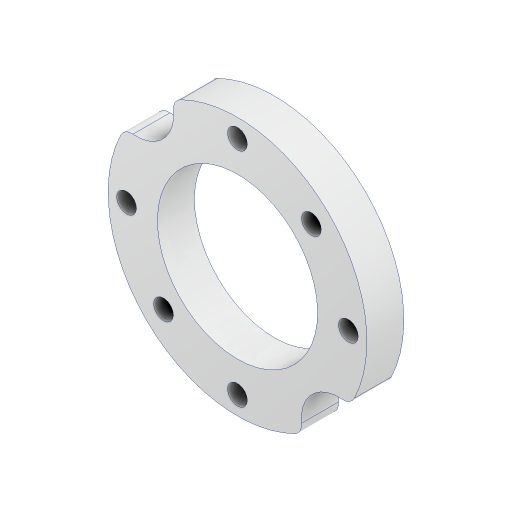
# Autodesk Inventor part: 큰기어 와셔
Saved by Autodesk Inventor 2023 (Build 270158000, 158)
## iProperties
Created: 2022-10-19
Part Number: 큰기어 와셔
Material: 알루미늄 6061
Document SubType Name: Modeling
Designer: PARK
Density: 2.7 g/cm^3
Appearance: 알루미늄 - 평지
Author: PARK
Autodesk Inventor part; units mm, degrees
ref_plane "YZ Plane" through (0, 0, 0) normal (1, 0, 0) x (0, 1, 0)
ref_plane "XZ Plane" through (0, 0, 0) normal (0, 1, 0) x (-1, 0, 0)
ref_plane "작업 평면1" through (168.9405, 113.6809, -210.8653) normal (0, 0, 1) x (-0.7019406, -0.7122354, 0)
sketch "스케치1" plane through (168.9405, 113.6809, -210.8653) normal (0, 0, 1) x (-0.7019406, -0.7122354, 0)
  circle A0 centre (0, -25.2484) radius 3 projected
  circle A1 centre (0, -2.2484) radius 13 projected
  circle A2 centre (-12.6349, 10.5718) radius 1.6 projected
  circle A3 centre (12.6349, -15.0687) radius 1.6 projected
  circle A4 centre (0.1235, 14.7217) radius 1.6 projected
  circle A5 centre (-0.1235, -19.2186) radius 1.6 projected
  circle A6 centre (-16.9701, -2.1249) radius 1.6 projected
  circle A7 centre (16.9701, -2.372) radius 1.6 projected
  circle A8 centre (12.8202, 10.3865) radius 1.6 projected
  circle A9 centre (-12.8202, -14.8834) radius 1.6 projected
  circle A10 centre (0, 20.7516) radius 3 projected
  arc A11 (-2.0317, -50.1272) -> (-0.57, -54.2453) centre (7.4248, -49.0892) ccw projected
  line L0 (0.57, -54.2453) -> (-0.57, -54.2453) projected
  arc A12 (0.57, -54.2453) -> (2.0317, -50.1272) centre (-7.4248, -49.0892) ccw projected
  arc A13 (2.5023, -49.6825) -> (2.0317, -50.1272) centre (2.5287, -50.1818) ccw projected
  arc A14 (2.5023, -49.6825) -> (3.4624, -49.6221) centre (0, -2.2484) ccw projected
  arc A15 (3.9852, -50.0043) -> (3.4624, -49.6221) centre (3.4989, -50.1207) ccw projected
  arc A16 (3.9852, -50.0043) -> (5.9514, -53.9067) centre (13.237, -47.7893) ccw projected
  line L1 (7.0824, -53.7639) -> (5.9514, -53.9067) projected
  arc A17 (7.0824, -53.7639) -> (8.0165, -49.4951) centre (-1.4956, -49.6504) ccw projected
  arc A18 (8.4277, -48.9948) -> (8.0165, -49.4951) centre (8.5164, -49.4869) ccw projected
  arc A19 (8.4277, -48.9948) -> (9.3726, -48.8146) centre (0, -2.2484) ccw projected
  arc A20 (9.9391, -49.1283) -> (9.3726, -48.8146) centre (9.4713, -49.3047) ccw projected
  arc A21 (9.9391, -49.1283) -> (12.379, -52.7535) centre (18.8404, -45.7711) ccw projected
  line L2 (13.4832, -52.47) -> (12.379, -52.7535) projected
  arc A22 (13.4832, -52.47) -> (13.8748, -48.1178) centre (4.4572, -49.4641) ccw projected
  arc A23 (14.2201, -47.5699) -> (13.8748, -48.1178) centre (14.3698, -48.047) ccw projected
  arc A24 (14.2201, -47.5699) -> (15.135, -47.2727) centre (0, -2.2484) ccw projected
  arc A25 (15.7364, -47.5129) -> (15.135, -47.2727) centre (15.2943, -47.7466) ccw projected
  arc A26 (15.7364, -47.5129) -> (18.6114, -50.8037) centre (24.1467, -43.0666) ccw projected
  line L3 (19.6713, -50.3841) -> (18.6114, -50.8037) projected
  arc A27 (19.6713, -50.3841) -> (19.5144, -46.0171) centre (10.3398, -48.5331) ccw projected
  arc A28 (19.7883, -45.4303) -> (19.5144, -46.0171) centre (19.9966, -45.8849) ccw projected
  arc A29 (19.7883, -45.4303) -> (20.6587, -45.0207) centre (0, -2.2484) ccw projected
  arc A30 (21.2854, -45.1837) -> (20.6587, -45.0207) centre (20.8762, -45.471) ccw projected
  arc A31 (21.2854, -45.1837) -> (24.5502, -48.0882) centre (29.0721, -39.7184) ccw projected
  line L4 (25.5492, -47.539) -> (24.5502, -48.0882) projected
  arc A32 (25.5492, -47.539) -> (24.8461, -43.2262) centre (16.0593, -46.8722) ccw projected
  arc A33 (25.0443, -42.6097) -> (24.8461, -43.2262) centre (25.308, -43.0345) ccw projected
  arc A34 (25.0443, -42.6097) -> (25.8566, -42.0942) centre (0, -2.2484) ccw projected
  arc A35 (26.4988, -42.1774) -> (25.8566, -42.0942) centre (26.1288, -42.5137) ccw projected
  arc A36 (26.4988, -42.1774) -> (30.1019, -44.6498) centre (33.5391, -35.7792) ccw projected
  line L5 (31.0241, -43.9798) -> (30.1019, -44.6498) projected
  arc A37 (31.0241, -43.9798) -> (29.7861, -39.789) centre (21.5255, -44.5076) ccw projected
  arc A38 (29.9055, -39.1525) -> (29.7861, -39.789) centre (30.2203, -39.541) ccw projected
  arc A39 (29.9055, -39.1525) -> (30.6467, -38.5393) centre (0, -2.2484) ccw projected
  arc A40 (31.2943, -38.5413) -> (30.6467, -38.5393) centre (30.9693, -38.9213) ccw projected
  arc A41 (31.2943, -38.5413) -> (35.1788, -40.5427) centre (37.4772, -31.3112) ccw projected
  line L6 (36.0098, -39.7623) -> (35.1788, -40.5427) projected
  arc A42 (36.0098, -39.7623) -> (34.2563, -35.7598) centre (26.6522, -41.4765) ccw projected
  arc A43 (34.295, -35.1134) -> (34.2563, -35.7598) centre (34.656, -35.4593) ccw projected
  arc A44 (34.295, -35.1134) -> (34.9535, -34.4121) centre (0, -2.2484) ccw projected
  arc A45 (35.5962, -34.333) -> (34.9535, -34.4121) centre (35.3214, -34.7507) ccw projected
  arc A46 (35.5962, -34.333) -> (39.7009, -35.8317) centre (40.8242, -26.3849) ccw projected
  line L7 (40.4276, -34.9533) -> (39.7009, -35.8317) projected
  arc A47 (40.4276, -34.9533) -> (38.1863, -31.2021) centre (31.3586, -37.8268) ccw projected
  arc A48 (38.1436, -30.5559) -> (38.1863, -31.2021) centre (38.5451, -30.8539) ccw projected
  arc A49 (38.1436, -30.5559) -> (38.7091, -29.7777) centre (0, -2.2484) ccw projected
  arc A50 (39.3368, -29.6186) -> (38.7091, -29.7777) centre (39.1165, -30.0674) ccw projected
  arc A51 (39.3368, -29.6186) -> (43.597, -30.591) centre (43.5274, -21.078) ccw projected
  line L8 (44.2078, -29.6285) -> (43.597, -30.591) projected
  arc A52 (44.2078, -29.6285) -> (41.514, -26.1878) centre (35.5705, -33.616) ccw projected
  arc A53 (41.3907, -25.5521) -> (41.514, -26.1878) centre (41.8264, -25.7974) ccw projected
  arc A54 (41.3907, -25.5521) -> (41.8542, -24.7091) centre (0, -2.2484) ccw projected
  arc A55 (42.457, -24.4725) -> (41.8542, -24.7091) centre (42.2947, -24.9455) ccw projected
  arc A56 (42.457, -24.4725) -> (46.8055, -24.9034) centre (45.5441, -15.4741) ccw projected
  line L9 (47.2909, -23.8719) -> (46.8055, -24.9034) projected
  arc A57 (47.2909, -23.8719) -> (44.1871, -20.7959) centre (39.2214, -28.9105) ccw projected
  arc A58 (43.985, -20.1807) -> (44.1871, -20.7959) centre (44.4481, -20.3694) ccw projected
  arc A59 (43.985, -20.1807) -> (44.3392, -19.2862) centre (0, -2.2484) ccw projected
  arc A60 (44.9076, -18.976) -> (44.3392, -19.2862) centre (44.8059, -19.4656) ccw projected
  arc A61 (44.9076, -18.976) -> (49.2758, -18.8585) centre (46.8426, -9.6616) ccw projected
  line L10 (49.6281, -17.7743) -> (49.2758, -18.8585) projected
  arc A62 (49.6281, -17.7743) -> (46.1633, -15.1116) centre (42.2538, -23.7845) ccw projected
  arc A63 (45.8857, -14.5265) -> (46.1633, -15.1116) centre (46.3687, -14.6557) ccw projected
  arc A64 (45.8857, -14.5265) -> (46.125, -13.5947) centre (0, -2.2484) ccw projected
  arc A65 (46.65, -13.2157) -> (46.125, -13.5947) centre (46.6105, -13.7141) ccw projected
  arc A66 (46.65, -13.2157) -> (50.9691, -12.5516) centre (47.4023, -3.7322) ccw projected
  line L11 (51.1827, -11.4318) -> (50.9691, -12.5516) projected
  arc A67 (51.1827, -11.4318) -> (47.4114, -9.2243) centre (44.6198, -18.3188) ccw projected
  arc A68 (47.0627, -8.6787) -> (47.4114, -9.2243) centre (47.5581, -8.7464) ccw projected
  arc A69 (47.0627, -8.6787) -> (47.1833, -7.7243) centre (0, -2.2484) ccw projected
  arc A70 (47.6567, -7.2824) -> (47.1833, -7.7243) centre (47.68, -7.7819) ccw projected
  arc A71 (47.6567, -7.2824) -> (51.8585, -6.0822) centre (47.2145, 2.2206) ccw projected
  line L12 (51.9301, -4.9445) -> (51.8585, -6.0822) projected
  arc A72 (51.9301, -4.9445) -> (47.9119, -3.2271) centre (46.2821, -12.5998) ccw projected
  arc A73 (47.4976, -2.7294) -> (47.9119, -3.2271) centre (47.9975, -2.7345) ccw projected
  arc A74 (47.4976, -2.7294) -> (47.4976, -1.7674) centre (0, -2.2484) ccw projected
  arc A75 (47.9119, -1.2698) -> (47.4976, -1.7674) centre (47.9975, -1.7624) ccw projected
  arc A76 (47.9119, -1.2698) -> (51.9301, 0.4476) centre (46.2821, 8.1029) ccw projected
  line L13 (51.8585, 1.5853) -> (51.9301, 0.4476) projected
  arc A77 (51.8585, 1.5853) -> (47.6567, 2.7856) centre (47.2145, -6.7175) ccw projected
  arc A78 (47.1833, 3.2274) -> (47.6567, 2.7856) centre (47.68, 3.285) ccw projected
  arc A79 (47.1833, 3.2274) -> (47.0627, 4.1818) centre (0, -2.2484) ccw projected
  arc A80 (47.4114, 4.7275) -> (47.0627, 4.1818) centre (47.5581, 4.2495) ccw projected
  arc A81 (47.4114, 4.7275) -> (51.1827, 6.9349) centre (44.6198, 13.822) ccw projected
  line L14 (50.9691, 8.0547) -> (51.1827, 6.9349) projected
  arc A82 (50.9691, 8.0547) -> (46.65, 8.7188) centre (47.4023, -0.7647) ccw projected
  arc A83 (46.125, 9.0978) -> (46.65, 8.7188) centre (46.6105, 9.2173) ccw projected
  arc A84 (46.125, 9.0978) -> (45.8857, 10.0296) centre (0, -2.2484) ccw projected
  arc A85 (46.1633, 10.6147) -> (45.8857, 10.0296) centre (46.3687, 10.1589) ccw projected
  arc A86 (46.1633, 10.6147) -> (49.6281, 13.2774) centre (42.2538, 19.2876) ccw projected
  line L15 (49.2758, 14.3616) -> (49.6281, 13.2774) projected
  arc A87 (49.2758, 14.3616) -> (44.9076, 14.4792) centre (46.8426, 5.1647) ccw projected
  arc A88 (44.3392, 14.7894) -> (44.9076, 14.4792) centre (44.8059, 14.9687) ccw projected
  arc A89 (44.3392, 14.7894) -> (43.985, 15.6838) centre (0, -2.2484) ccw projected
  arc A90 (44.1871, 16.299) -> (43.985, 15.6838) centre (44.4481, 15.8726) ccw projected
  arc A91 (44.1871, 16.299) -> (47.2909, 19.375) centre (39.2214, 24.4136) ccw projected
  line L16 (46.8055, 20.4065) -> (47.2909, 19.375) projected
  arc A92 (46.8055, 20.4065) -> (42.457, 19.9757) centre (45.5441, 10.9772) ccw projected
  arc A93 (41.8542, 20.2122) -> (42.457, 19.9757) centre (42.2947, 20.4486) ccw projected
  arc A94 (41.8542, 20.2122) -> (41.3907, 21.0552) centre (0, -2.2484) ccw projected
  arc A95 (41.514, 21.6909) -> (41.3907, 21.0552) centre (41.8264, 21.3005) ccw projected
  arc A96 (41.514, 21.6909) -> (44.2078, 25.1316) centre (35.5705, 29.1191) ccw projected
  line L17 (43.597, 26.0941) -> (44.2078, 25.1316) projected
  arc A97 (43.597, 26.0941) -> (39.3368, 25.1217) centre (43.5274, 16.5811) ccw projected
  arc A98 (38.7091, 25.2808) -> (39.3368, 25.1217) centre (39.1165, 25.5706) ccw projected
  arc A99 (38.7091, 25.2808) -> (38.1436, 26.0591) centre (0, -2.2484) ccw projected
  arc A100 (38.1863, 26.7052) -> (38.1436, 26.0591) centre (38.5451, 26.357) ccw projected
  arc A101 (38.1863, 26.7052) -> (40.4276, 30.4564) centre (31.3586, 33.3299) ccw projected
  line L18 (39.7009, 31.3348) -> (40.4276, 30.4564) projected
  arc A102 (39.7009, 31.3348) -> (35.5962, 29.8361) centre (40.8242, 21.888) ccw projected
  arc A103 (34.9535, 29.9152) -> (35.5962, 29.8361) centre (35.3214, 30.2538) ccw projected
  arc A104 (34.9535, 29.9152) -> (34.295, 30.6165) centre (0, -2.2484) ccw projected
  arc A105 (34.2563, 31.2629) -> (34.295, 30.6165) centre (34.656, 30.9625) ccw projected
  arc A106 (34.2563, 31.2629) -> (36.0098, 35.2655) centre (26.6522, 36.9797) ccw projected
  line L19 (35.1788, 36.0458) -> (36.0098, 35.2655) projected
  arc A107 (35.1788, 36.0458) -> (31.2943, 34.0445) centre (37.4772, 26.8143) ccw projected
  arc A108 (30.6467, 34.0425) -> (31.2943, 34.0445) centre (30.9693, 34.4245) ccw projected
  arc A109 (30.6467, 34.0425) -> (29.9055, 34.6557) centre (0, -2.2484) ccw projected
  arc A110 (29.7861, 35.2921) -> (29.9055, 34.6557) centre (30.2203, 35.0441) ccw projected
  arc A111 (29.7861, 35.2921) -> (31.0241, 39.4829) centre (21.5255, 40.0107) ccw projected
  line L20 (30.1019, 40.153) -> (31.0241, 39.4829) projected
  arc A112 (30.1019, 40.153) -> (26.4988, 37.6805) centre (33.5391, 31.2823) ccw projected
  arc A113 (25.8566, 37.5973) -> (26.4988, 37.6805) centre (26.1288, 38.0168) ccw projected
  arc A114 (25.8566, 37.5973) -> (25.0443, 38.1128) centre (0, -2.2484) ccw projected
  arc A115 (24.8461, 38.7293) -> (25.0443, 38.1128) centre (25.308, 38.5377) ccw projected
  arc A116 (24.8461, 38.7293) -> (25.5492, 43.0422) centre (16.0593, 42.3754) ccw projected
  line L21 (24.5502, 43.5914) -> (25.5492, 43.0422) projected
  arc A117 (24.5502, 43.5914) -> (21.2854, 40.6868) centre (29.0721, 35.2215) ccw projected
  arc A118 (20.6587, 40.5238) -> (21.2854, 40.6868) centre (20.8762, 40.9741) ccw projected
  arc A119 (20.6587, 40.5238) -> (19.7883, 40.9334) centre (0, -2.2484) ccw projected
  arc A120 (19.5144, 41.5202) -> (19.7883, 40.9334) centre (19.9966, 41.388) ccw projected
  arc A121 (19.5144, 41.5202) -> (19.6713, 45.8872) centre (10.3398, 44.0363) ccw projected
  line L22 (18.6114, 46.3069) -> (19.6713, 45.8872) projected
  arc A122 (18.6114, 46.3069) -> (15.7364, 43.016) centre (24.1467, 38.5697) ccw projected
  arc A123 (15.135, 42.7758) -> (15.7364, 43.016) centre (15.2943, 43.2497) ccw projected
  arc A124 (15.135, 42.7758) -> (14.2201, 43.0731) centre (0, -2.2484) ccw projected
  arc A125 (13.8748, 43.6209) -> (14.2201, 43.0731) centre (14.3698, 43.5501) ccw projected
  arc A126 (13.8748, 43.6209) -> (13.4832, 47.9731) centre (4.4572, 44.9672) ccw projected
  line L23 (12.379, 48.2566) -> (13.4832, 47.9731) projected
  arc A127 (12.379, 48.2566) -> (9.9391, 44.6314) centre (18.8404, 41.2742) ccw projected
  arc A128 (9.3726, 44.3177) -> (9.9391, 44.6314) centre (9.4713, 44.8079) ccw projected
  arc A129 (9.3726, 44.3177) -> (8.4277, 44.4979) centre (0, -2.2484) ccw projected
  arc A130 (8.0165, 44.9982) -> (8.4277, 44.4979) centre (8.5164, 44.99) ccw projected
  arc A131 (8.0165, 44.9982) -> (7.0824, 49.267) centre (-1.4956, 45.1535) ccw projected
  line L24 (5.9514, 49.4099) -> (7.0824, 49.267) projected
  arc A132 (5.9514, 49.4099) -> (3.9852, 45.5074) centre (13.237, 43.2924) ccw projected
  arc A133 (3.4624, 45.1252) -> (3.9852, 45.5074) centre (3.4989, 45.6239) ccw projected
  arc A134 (3.4624, 45.1252) -> (2.5023, 45.1856) centre (0, -2.2484) ccw projected
  arc A135 (2.0317, 45.6304) -> (2.5023, 45.1856) centre (2.5287, 45.6849) ccw projected
  arc A136 (2.0317, 45.6304) -> (0.57, 49.7484) centre (-7.4248, 44.5923) ccw projected
  line L25 (-0.57, 49.7484) -> (0.57, 49.7484) projected
  arc A137 (-0.57, 49.7484) -> (-2.0317, 45.6304) centre (7.4248, 44.5923) ccw projected
  arc A138 (-2.5023, 45.1856) -> (-2.0317, 45.6304) centre (-2.5287, 45.6849) ccw projected
  arc A139 (-2.5023, 45.1856) -> (-3.4624, 45.1252) centre (0, -2.2484) ccw projected
  arc A140 (-3.9852, 45.5074) -> (-3.4624, 45.1252) centre (-3.4989, 45.6239) ccw projected
  arc A141 (-3.9852, 45.5074) -> (-5.9514, 49.4099) centre (-13.237, 43.2924) ccw projected
  line L26 (-7.0824, 49.267) -> (-5.9514, 49.4099) projected
  arc A142 (-7.0824, 49.267) -> (-8.0165, 44.9982) centre (1.4956, 45.1535) ccw projected
  arc A143 (-8.4277, 44.4979) -> (-8.0165, 44.9982) centre (-8.5164, 44.99) ccw projected
  arc A144 (-8.4277, 44.4979) -> (-9.3726, 44.3177) centre (0, -2.2484) ccw projected
  arc A145 (-9.9391, 44.6314) -> (-9.3726, 44.3177) centre (-9.4713, 44.8079) ccw projected
  arc A146 (-9.9391, 44.6314) -> (-12.379, 48.2566) centre (-18.8404, 41.2742) ccw projected
  line L27 (-13.4832, 47.9731) -> (-12.379, 48.2566) projected
  arc A147 (-13.4832, 47.9731) -> (-13.8748, 43.6209) centre (-4.4572, 44.9672) ccw projected
  arc A148 (-14.2201, 43.0731) -> (-13.8748, 43.6209) centre (-14.3698, 43.5501) ccw projected
  arc A149 (-14.2201, 43.0731) -> (-15.135, 42.7758) centre (0, -2.2484) ccw projected
  arc A150 (-15.7364, 43.016) -> (-15.135, 42.7758) centre (-15.2943, 43.2497) ccw projected
  arc A151 (-15.7364, 43.016) -> (-18.6114, 46.3069) centre (-24.1467, 38.5697) ccw projected
  line L28 (-19.6713, 45.8872) -> (-18.6114, 46.3069) projected
  arc A152 (-19.6713, 45.8872) -> (-19.5144, 41.5202) centre (-10.3398, 44.0363) ccw projected
  arc A153 (-19.7883, 40.9334) -> (-19.5144, 41.5202) centre (-19.9966, 41.388) ccw projected
  arc A154 (-19.7883, 40.9334) -> (-20.6587, 40.5238) centre (0, -2.2484) ccw projected
  arc A155 (-21.2854, 40.6868) -> (-20.6587, 40.5238) centre (-20.8762, 40.9741) ccw projected
  arc A156 (-21.2854, 40.6868) -> (-24.5502, 43.5914) centre (-29.0721, 35.2215) ccw projected
  line L29 (-25.5492, 43.0422) -> (-24.5502, 43.5914) projected
  arc A157 (-25.5492, 43.0422) -> (-24.8461, 38.7293) centre (-16.0593, 42.3754) ccw projected
  arc A158 (-25.0443, 38.1128) -> (-24.8461, 38.7293) centre (-25.308, 38.5377) ccw projected
  arc A159 (-25.0443, 38.1128) -> (-25.8566, 37.5973) centre (0, -2.2484) ccw projected
  arc A160 (-26.4988, 37.6805) -> (-25.8566, 37.5973) centre (-26.1288, 38.0168) ccw projected
  arc A161 (-26.4988, 37.6805) -> (-30.1019, 40.153) centre (-33.5391, 31.2823) ccw projected
  line L30 (-31.0241, 39.4829) -> (-30.1019, 40.153) projected
  arc A162 (-31.0241, 39.4829) -> (-29.7861, 35.2921) centre (-21.5255, 40.0107) ccw projected
  arc A163 (-29.9055, 34.6557) -> (-29.7861, 35.2921) centre (-30.2203, 35.0441) ccw projected
  arc A164 (-29.9055, 34.6557) -> (-30.6467, 34.0425) centre (0, -2.2484) ccw projected
  arc A165 (-31.2943, 34.0445) -> (-30.6467, 34.0425) centre (-30.9693, 34.4245) ccw projected
  arc A166 (-31.2943, 34.0445) -> (-35.1788, 36.0458) centre (-37.4772, 26.8143) ccw projected
  line L31 (-36.0098, 35.2655) -> (-35.1788, 36.0458) projected
  arc A167 (-36.0098, 35.2655) -> (-34.2563, 31.2629) centre (-26.6522, 36.9797) ccw projected
  arc A168 (-34.295, 30.6165) -> (-34.2563, 31.2629) centre (-34.656, 30.9625) ccw projected
  arc A169 (-34.295, 30.6165) -> (-34.9535, 29.9152) centre (0, -2.2484) ccw projected
  arc A170 (-35.5962, 29.8361) -> (-34.9535, 29.9152) centre (-35.3214, 30.2538) ccw projected
  arc A171 (-35.5962, 29.8361) -> (-39.7009, 31.3348) centre (-40.8242, 21.888) ccw projected
  line L32 (-40.4276, 30.4564) -> (-39.7009, 31.3348) projected
  arc A172 (-40.4276, 30.4564) -> (-38.1863, 26.7052) centre (-31.3586, 33.3299) ccw projected
  arc A173 (-38.1436, 26.0591) -> (-38.1863, 26.7052) centre (-38.5451, 26.357) ccw projected
  arc A174 (-38.1436, 26.0591) -> (-38.7091, 25.2808) centre (0, -2.2484) ccw projected
  arc A175 (-39.3368, 25.1217) -> (-38.7091, 25.2808) centre (-39.1165, 25.5706) ccw projected
  arc A176 (-39.3368, 25.1217) -> (-43.597, 26.0941) centre (-43.5274, 16.5811) ccw projected
  line L33 (-44.2078, 25.1316) -> (-43.597, 26.0941) projected
  arc A177 (-44.2078, 25.1316) -> (-41.514, 21.6909) centre (-35.5705, 29.1191) ccw projected
  arc A178 (-41.3907, 21.0552) -> (-41.514, 21.6909) centre (-41.8264, 21.3005) ccw projected
  arc A179 (-41.3907, 21.0552) -> (-41.8542, 20.2122) centre (0, -2.2484) ccw projected
  arc A180 (-42.457, 19.9757) -> (-41.8542, 20.2122) centre (-42.2947, 20.4486) ccw projected
  arc A181 (-42.457, 19.9757) -> (-46.8055, 20.4065) centre (-45.5441, 10.9772) ccw projected
  line L34 (-47.2909, 19.375) -> (-46.8055, 20.4065) projected
  arc A182 (-47.2909, 19.375) -> (-44.1871, 16.299) centre (-39.2214, 24.4136) ccw projected
  arc A183 (-43.985, 15.6838) -> (-44.1871, 16.299) centre (-44.4481, 15.8726) ccw projected
  arc A184 (-43.985, 15.6838) -> (-44.3392, 14.7894) centre (0, -2.2484) ccw projected
  arc A185 (-44.9076, 14.4792) -> (-44.3392, 14.7894) centre (-44.8059, 14.9687) ccw projected
  arc A186 (-44.9076, 14.4792) -> (-49.2758, 14.3616) centre (-46.8426, 5.1647) ccw projected
  line L35 (-49.6281, 13.2774) -> (-49.2758, 14.3616) projected
  arc A187 (-49.6281, 13.2774) -> (-46.1633, 10.6147) centre (-42.2538, 19.2876) ccw projected
  arc A188 (-45.8857, 10.0296) -> (-46.1633, 10.6147) centre (-46.3687, 10.1589) ccw projected
  arc A189 (-45.8857, 10.0296) -> (-46.125, 9.0978) centre (0, -2.2484) ccw projected
  arc A190 (-46.65, 8.7188) -> (-46.125, 9.0978) centre (-46.6105, 9.2173) ccw projected
  arc A191 (-46.65, 8.7188) -> (-50.9691, 8.0547) centre (-47.4023, -0.7647) ccw projected
  line L36 (-51.1827, 6.9349) -> (-50.9691, 8.0547) projected
  arc A192 (-51.1827, 6.9349) -> (-47.4114, 4.7275) centre (-44.6198, 13.822) ccw projected
  arc A193 (-47.0627, 4.1818) -> (-47.4114, 4.7275) centre (-47.5581, 4.2495) ccw projected
  arc A194 (-47.0627, 4.1818) -> (-47.1833, 3.2274) centre (0, -2.2484) ccw projected
  arc A195 (-47.6567, 2.7856) -> (-47.1833, 3.2274) centre (-47.68, 3.285) ccw projected
  arc A196 (-47.6567, 2.7856) -> (-51.8585, 1.5853) centre (-47.2145, -6.7175) ccw projected
  line L37 (-51.9301, 0.4476) -> (-51.8585, 1.5853) projected
  arc A197 (-51.9301, 0.4476) -> (-47.9119, -1.2698) centre (-46.2821, 8.1029) ccw projected
  arc A198 (-47.4976, -1.7674) -> (-47.9119, -1.2698) centre (-47.9975, -1.7624) ccw projected
  arc A199 (-47.4976, -1.7674) -> (-47.4976, -2.7294) centre (0, -2.2484) ccw projected
  arc A200 (-47.9119, -3.2271) -> (-47.4976, -2.7294) centre (-47.9975, -2.7345) ccw projected
  arc A201 (-47.9119, -3.2271) -> (-51.9301, -4.9445) centre (-46.2821, -12.5998) ccw projected
  line L38 (-51.8585, -6.0822) -> (-51.9301, -4.9445) projected
  arc A202 (-51.8585, -6.0822) -> (-47.6567, -7.2824) centre (-47.2145, 2.2206) ccw projected
  arc A203 (-47.1833, -7.7243) -> (-47.6567, -7.2824) centre (-47.68, -7.7819) ccw projected
  arc A204 (-47.1833, -7.7243) -> (-47.0627, -8.6787) centre (0, -2.2484) ccw projected
  arc A205 (-47.4114, -9.2243) -> (-47.0627, -8.6787) centre (-47.5581, -8.7464) ccw projected
  arc A206 (-47.4114, -9.2243) -> (-51.1827, -11.4318) centre (-44.6198, -18.3188) ccw projected
  line L39 (-50.9691, -12.5516) -> (-51.1827, -11.4318) projected
  arc A207 (-50.9691, -12.5516) -> (-46.65, -13.2157) centre (-47.4023, -3.7322) ccw projected
  arc A208 (-46.125, -13.5947) -> (-46.65, -13.2157) centre (-46.6105, -13.7141) ccw projected
  arc A209 (-46.125, -13.5947) -> (-45.8857, -14.5265) centre (0, -2.2484) ccw projected
  arc A210 (-46.1633, -15.1116) -> (-45.8857, -14.5265) centre (-46.3687, -14.6557) ccw projected
  arc A211 (-46.1633, -15.1116) -> (-49.6281, -17.7743) centre (-42.2538, -23.7845) ccw projected
  line L40 (-49.2758, -18.8585) -> (-49.6281, -17.7743) projected
  arc A212 (-49.2758, -18.8585) -> (-44.9076, -18.976) centre (-46.8426, -9.6616) ccw projected
  arc A213 (-44.3392, -19.2862) -> (-44.9076, -18.976) centre (-44.8059, -19.4656) ccw projected
  arc A214 (-44.3392, -19.2862) -> (-43.985, -20.1807) centre (0, -2.2484) ccw projected
  arc A215 (-44.1871, -20.7959) -> (-43.985, -20.1807) centre (-44.4481, -20.3694) ccw projected
  arc A216 (-44.1871, -20.7959) -> (-47.2909, -23.8719) centre (-39.2214, -28.9105) ccw projected
  line L41 (-46.8055, -24.9034) -> (-47.2909, -23.8719) projected
  arc A217 (-46.8055, -24.9034) -> (-42.457, -24.4725) centre (-45.5441, -15.4741) ccw projected
  arc A218 (-41.8542, -24.7091) -> (-42.457, -24.4725) centre (-42.2947, -24.9455) ccw projected
  arc A219 (-41.8542, -24.7091) -> (-41.3907, -25.5521) centre (0, -2.2484) ccw projected
  arc A220 (-41.514, -26.1878) -> (-41.3907, -25.5521) centre (-41.8264, -25.7974) ccw projected
  arc A221 (-41.514, -26.1878) -> (-44.2078, -29.6285) centre (-35.5705, -33.616) ccw projected
  line L42 (-43.597, -30.591) -> (-44.2078, -29.6285) projected
  arc A222 (-43.597, -30.591) -> (-39.3368, -29.6186) centre (-43.5274, -21.078) ccw projected
  arc A223 (-38.7091, -29.7777) -> (-39.3368, -29.6186) centre (-39.1165, -30.0674) ccw projected
  arc A224 (-38.7091, -29.7777) -> (-38.1436, -30.5559) centre (0, -2.2484) ccw projected
  arc A225 (-38.1863, -31.2021) -> (-38.1436, -30.5559) centre (-38.5451, -30.8539) ccw projected
  arc A226 (-38.1863, -31.2021) -> (-40.4276, -34.9533) centre (-31.3586, -37.8268) ccw projected
  line L43 (-39.7009, -35.8317) -> (-40.4276, -34.9533) projected
  arc A227 (-39.7009, -35.8317) -> (-35.5962, -34.333) centre (-40.8242, -26.3849) ccw projected
  arc A228 (-34.9535, -34.4121) -> (-35.5962, -34.333) centre (-35.3214, -34.7507) ccw projected
  arc A229 (-34.9535, -34.4121) -> (-34.295, -35.1134) centre (0, -2.2484) ccw projected
  arc A230 (-34.2563, -35.7598) -> (-34.295, -35.1134) centre (-34.656, -35.4593) ccw projected
  arc A231 (-34.2563, -35.7598) -> (-36.0098, -39.7623) centre (-26.6522, -41.4765) ccw projected
  line L44 (-35.1788, -40.5427) -> (-36.0098, -39.7623) projected
  arc A232 (-35.1788, -40.5427) -> (-31.2943, -38.5413) centre (-37.4772, -31.3112) ccw projected
  arc A233 (-30.6467, -38.5393) -> (-31.2943, -38.5413) centre (-30.9693, -38.9213) ccw projected
  arc A234 (-30.6467, -38.5393) -> (-29.9055, -39.1525) centre (0, -2.2484) ccw projected
  arc A235 (-29.7861, -39.789) -> (-29.9055, -39.1525) centre (-30.2203, -39.541) ccw projected
  arc A236 (-29.7861, -39.789) -> (-31.0241, -43.9798) centre (-21.5255, -44.5076) ccw projected
  line L45 (-30.1019, -44.6498) -> (-31.0241, -43.9798) projected
  arc A237 (-30.1019, -44.6498) -> (-26.4988, -42.1774) centre (-33.5391, -35.7792) ccw projected
  arc A238 (-25.8566, -42.0942) -> (-26.4988, -42.1774) centre (-26.1288, -42.5137) ccw projected
  arc A239 (-25.8566, -42.0942) -> (-25.0443, -42.6097) centre (0, -2.2484) ccw projected
  arc A240 (-24.8461, -43.2262) -> (-25.0443, -42.6097) centre (-25.308, -43.0345) ccw projected
  arc A241 (-24.8461, -43.2262) -> (-25.5492, -47.539) centre (-16.0593, -46.8722) ccw projected
  line L46 (-24.5502, -48.0882) -> (-25.5492, -47.539) projected
  arc A242 (-24.5502, -48.0882) -> (-21.2854, -45.1837) centre (-29.0721, -39.7184) ccw projected
  arc A243 (-20.6587, -45.0207) -> (-21.2854, -45.1837) centre (-20.8762, -45.471) ccw projected
  arc A244 (-20.6587, -45.0207) -> (-19.7883, -45.4303) centre (0, -2.2484) ccw projected
  arc A245 (-19.5144, -46.0171) -> (-19.7883, -45.4303) centre (-19.9966, -45.8849) ccw projected
  arc A246 (-19.5144, -46.0171) -> (-19.6713, -50.3841) centre (-10.3398, -48.5331) ccw projected
  line L47 (-18.6114, -50.8037) -> (-19.6713, -50.3841) projected
  arc A247 (-18.6114, -50.8037) -> (-15.7364, -47.5129) centre (-24.1467, -43.0666) ccw projected
  arc A248 (-15.135, -47.2727) -> (-15.7364, -47.5129) centre (-15.2943, -47.7466) ccw projected
  arc A249 (-15.135, -47.2727) -> (-14.2201, -47.5699) centre (0, -2.2484) ccw projected
  arc A250 (-13.8748, -48.1178) -> (-14.2201, -47.5699) centre (-14.3698, -48.047) ccw projected
  arc A251 (-13.8748, -48.1178) -> (-13.4832, -52.47) centre (-4.4572, -49.4641) ccw projected
  line L48 (-12.379, -52.7535) -> (-13.4832, -52.47) projected
  arc A252 (-12.379, -52.7535) -> (-9.9391, -49.1283) centre (-18.8404, -45.7711) ccw projected
  arc A253 (-9.3726, -48.8146) -> (-9.9391, -49.1283) centre (-9.4713, -49.3047) ccw projected
  arc A254 (-9.3726, -48.8146) -> (-8.4277, -48.9948) centre (0, -2.2484) ccw projected
  arc A255 (-8.0165, -49.4951) -> (-8.4277, -48.9948) centre (-8.5164, -49.4869) ccw projected
  arc A256 (-8.0165, -49.4951) -> (-7.0824, -53.7639) centre (1.4956, -49.6504) ccw projected
  line L49 (-5.9514, -53.9067) -> (-7.0824, -53.7639) projected
  arc A257 (-5.9514, -53.9067) -> (-3.9852, -50.0043) centre (-13.237, -47.7893) ccw projected
  arc A258 (-3.4624, -49.6221) -> (-3.9852, -50.0043) centre (-3.4989, -50.1207) ccw projected
  arc A259 (-3.4624, -49.6221) -> (-2.5023, -49.6825) centre (0, -2.2484) ccw projected
  arc A260 (-2.0317, -50.1272) -> (-2.5023, -49.6825) centre (-2.5287, -50.1818) ccw projected
  circle A261 centre (0, -2.2484) radius 21
  circle A262 centre (0, 20.7516) radius 6.0312
  circle A263 centre (0, -25.2484) radius 6.0312
  point P0 (-5.3911, -22.5446)
  point P1 (5.3911, -22.5446)
  point P2 (5.3911, 18.0478)
  point P3 (-5.3911, 18.0478)
  dimension "d0" = 42
  constraints: 3 coincident, 1 centre point, 6 other
  measures "d0" diameter of A261
extrude "돌출1" add sketch "스케치1" along normal blind 5 contours A263 A5 A261 A262 A4 | A263 A5 | A262 A4 picked at (-0.1641, -18.7025) picked at (0.0932, 14.205)
fillet "모깎기1" radius 2 4 edges at (185.5791, 104.8522, -208.3653) (178.0106, 97.1727, -208.3653) (149.0992, 125.6661, -208.3653) (156.6677, 133.3456, -208.3653)
sketch "스케치2" plane through (168.9405, 113.6809, -205.8653) normal (0, 0, 1) x (0.7122354, -0.7019406, 0)
  arc A0 (-22.0831, 6.8982) -> (-21.4528, 4.687) centre (-20.1941, 6.2412) ccw projected
  arc A1 (-21.4528, -4.687) -> (-21.4528, 4.687) centre (-25.2484, 0) ccw projected
  arc A2 (-21.4528, -4.687) -> (-22.0831, -6.8982) centre (-20.1941, -6.2412) ccw projected
  arc A3 (-22.0831, -6.8982) -> (17.5862, -6.8982) centre (-2.2484, 0) ccw projected
  arc A4 (17.5862, -6.8982) -> (16.9559, -4.687) centre (15.6972, -6.2412) ccw projected
  arc A5 (16.9559, 4.687) -> (16.9559, -4.687) centre (20.7516, 0) ccw projected
  arc A6 (16.9559, 4.687) -> (17.5862, 6.8982) centre (15.6972, 6.2412) ccw projected
  arc A7 (17.5862, 6.8982) -> (-22.0831, 6.8982) centre (-2.2484, 0) ccw projected
  circle A8 centre (-14.8834, 12.8202) radius 1.6 projected
  circle A9 centre (10.3865, -12.8202) radius 1.6 projected
  circle A10 centre (-2.372, -16.9701) radius 1.6 projected
  circle A11 centre (-2.1249, 16.9701) radius 1.6 projected
  circle A12 centre (-15.0687, -12.6349) radius 1.6 projected
  circle A13 centre (10.5718, 12.6349) radius 1.6 projected
  circle A14 centre (-2.2484, 0) radius 13 projected
extrude "돌출2" add sketch "스케치2" along normal blind 1
